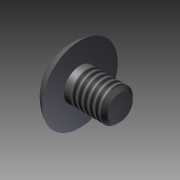
# Autodesk Inventor part: BOX-TRSS4-5
Saved by Autodesk Inventor 2011 SP1 (Build 150282100, 282)
## iProperties
Created: 2015-02-01
Part Number: BOX-TRSS4-5
Catalog Web Link: www.cadenas.de
Description: BOX-TRSS-(Box Set) Cross Recessed Truss Machine Screws
Vendor: MISUMI
Document SubType Name: Modeling
Designer: psAdmin
Manufacturer: MISUMI
Mass: 0.154361 g
Surface Area: 2.40929 cm^2
Volume: 0.154361 cm^3
Density: 1 g/cm^3
Category: PARTsolutions
Company: MISUMI
Title: BOX-TRSS4-5
Author: Cadenas PARTsolutions
Comments: (Box Set) Cross Recessed Truss Machine Screws
PSOL_IDENT_0: {\\10.0.0.236\data_v8\23d-libs\misumi\metric\27_screws_nuts\box_trss.prj},167 {VTYP=3D},{NB=BOX-TRSS
PSOL_IDENT_1: 4-5},{LINA=BOX-TRSS4-5},{NN=BOX-TRSS},{DATE=17.11.2014 07:43:32},{GEOMDATE=25.03.2010 00:00:00},{VER
PSOL_IDENT_2: SION=},{LINEID=60},{LINESUBID=-1},{WBVAR=L}  {NB=BOX-TRSS4-5},{LINA=BOX-TRSS4-5},{KT=DUMMY},{PN=BOX-
PSOL_IDENT_3: TRSS4-5},{TYPE=BOX-TRSS},{MAT=304 Stainless Steel },{M1=4},{M=4.0},{L=5},{L0=5,6,8,10},{MP=4x0.7},{A=
PSOL_IDENT_4: 9.4},{E=2.5},{PCS=1000 pcs.}
SUPPLIER: MISUMI
ARTICLENO: BOX-TRSS4-5
BOMINFO: BOX-TRSS4-5
CREATOR: CADENAS GmbH
Autodesk Inventor part; units mm, degrees
sketch "Sketch_1" plane through (0, 0, 0) normal (0, 0, 1) x (1, 0, 0)
  line L0 (5, 0) -> (-2.5, 0)
  line L1 (-2.5, 0) -> (-2.5, 0.94)
  arc A0 (0, 4.7) -> (-2.5, 0.94) centre (2.1827, 0.5376) ccw
  line L2 (0, 4.7) -> (0, 2)
  line L3 (0, 2) -> (4.5705, 2)
  line L4 (4.5705, 2) -> (5, 1.5705)
  line L5 (5, 1.5705) -> (5, 0)
  line L6 (5, 0) -> (-2.5, 0)
  constraints: 14 end point, 2 point on circle, 1 centre point
revolve "Revolution1" add sketch "Sketch_1" angle 360 about axis through (5, 0, 0) along (1, 0, 0)
thread "Thread1" size "M4x0.7" class "6g" standard "ISO Metric profile" length 4.2 offset 0.8
sketch "Sketch_2" plane through (-2.5, 0, 0) normal (1, 0, 0) x (0, 0, -1)
  line L0 (-2.35, 0.6267) -> (-2.35, -0.6267)
  line L1 (-2.35, -0.6267) -> (-0.6267, -0.6267)
  line L2 (-0.6267, -0.6267) -> (-0.6267, -2.35)
  line L3 (-0.6267, -2.35) -> (0.6267, -2.35)
  line L4 (0.6267, -2.35) -> (0.6267, -0.6267)
  line L5 (0.6267, -0.6267) -> (2.35, -0.6267)
  line L6 (2.35, -0.6267) -> (2.35, 0.6267)
  line L7 (2.35, 0.6267) -> (0.6267, 0.6267)
  line L8 (0.6267, 0.6267) -> (0.6267, 2.35)
  line L9 (0.6267, 2.35) -> (-0.6267, 2.35)
  line L10 (-0.6267, 2.35) -> (-0.6267, 0.6267)
  line L11 (-0.6267, 0.6267) -> (-2.35, 0.6267)
  constraints: 24 end point
extrude "Extrusion1" cut sketch "Sketch_2" along normal mid plane 2.5
ref_plane "bolt_to_parts_XY" through (0, 0, 0) normal (1, 0, 0) x (0, 0, -1)
ref_plane "bolt_to_parts_YZ" through (0, 0, 0) normal (0, 0, -1) x (0, 1, 0)
ref_plane "bolt_to_parts_ZX" through (0, 0, 0) normal (0, 1, 0) x (1, 0, 0)
body "Solid1"
